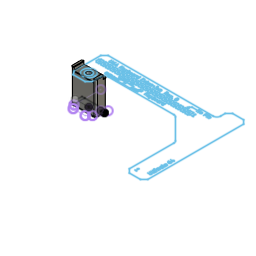
U64_KeybExt_Support v2 (Autodesk Fusion 360 design; units mm, degrees)
Autodesk Fusion 360 part; units mm, degrees
ref_plane "WorkPlane1" through (0, 0, 16) normal (0, 0, 1) x (1, 0, 0) in component "PCB"
sketch "U64_KB_Ada" plane through (0, 0, 16) normal (0, 0, 1) x (1, 0, 0) in component "PCB"
  line L0 (47.6716, 39.5) -> (12, 39.5)
  line L1 (71, 2) -> (71, 54)
  arc A0 (61, 26.1716) -> (60.4142, 27.5858) centre (59, 26.1716) ccw
  arc A1 (59, 49.5) -> (61, 51.5) centre (59, 51.5) ccw
  line L2 (71, 54) -> (69, 56)
  arc A2 (12, 39.5) -> (10, 37.5) centre (12, 37.5) ccw
  line L3 (61, 2) -> (63, 0)
  line L4 (0, 33) -> (0, 47.5)
  line L5 (61, 26.1716) -> (61, 2)
  line L6 (59, 49.5) -> (2, 49.5)
  line L7 (2, 49.5) -> (0, 47.5)
  line L8 (1.5, 31) -> (0, 33)
  line L9 (69, 0) -> (71, 2)
  line L10 (63, 0) -> (69, 0)
  line L11 (61, 54) -> (61, 51.5)
  line L12 (10, 33) -> (8, 31)
  line L13 (69, 56) -> (63, 56)
  line L14 (63, 56) -> (61, 54)
  line L15 (10, 37.5) -> (10, 33)
  line L16 (49.0858, 38.9142) -> (60.4142, 27.5858)
  arc A3 (49.0858, 38.9142) -> (47.6716, 39.5) centre (47.6716, 37.5) ccw
  line L17 (8, 31) -> (1.5, 31)
  line L18 (21.59, 45.135) -> (22.225, 45.77)
  line L19 (15.875, 43.23) -> (14.605, 43.23)
  line L20 (17.145, 45.77) -> (18.415, 45.77)
  line L21 (21.59, 45.135) -> (20.955, 45.77)
  line L22 (13.97, 45.135) -> (13.335, 45.77)
  line L23 (5.715, 43.23) -> (6.35, 43.865)
  line L24 (9.525, 43.23) -> (8.89, 43.865)
  line L25 (13.204, 40.1285) -> (13.5992, 41.215)
  line L26 (9.525, 45.77) -> (10.795, 45.77)
  line L27 (21.59, 43.865) -> (21.59, 45.135)
  line L28 (20.955, 43.23) -> (21.59, 43.865)
  line L29 (11.43, 43.865) -> (10.795, 43.23)
  line L30 (6.985, 45.77) -> (8.255, 45.77)
  line L31 (6.35, 43.865) -> (6.35, 45.135)
  line L32 (13.97, 43.865) -> (13.97, 45.135)
  line L33 (11.43, 45.135) -> (12.065, 45.77)
  line L34 (12.065, 43.23) -> (11.43, 43.865)
  circle A4 centre (5, 36) radius 3.1789
  circle A5 centre (5, 36) radius 1.7463
  line L35 (13.97, 45.135) -> (14.605, 45.77)
  line L36 (4.445, 43.23) -> (3.81, 43.865)
  line L37 (16.51, 43.865) -> (15.875, 43.23)
  line L38 (16.51, 43.865) -> (16.51, 45.135)
  line L39 (20.955, 43.23) -> (19.685, 43.23)
  line L40 (8.89, 45.135) -> (9.525, 45.77)
  line L41 (12.065, 45.77) -> (13.335, 45.77)
  line L42 (19.685, 45.77) -> (20.955, 45.77)
  line L43 (19.685, 43.23) -> (19.05, 43.865)
  line L44 (10.795, 43.23) -> (9.525, 43.23)
  line L45 (27.305, 43.23) -> (26.67, 43.865)
  line L46 (19.05, 43.865) -> (19.05, 45.135)
  line L47 (23.495, 45.77) -> (24.13, 45.135)
  line L48 (14.605, 45.77) -> (15.875, 45.77)
  line L49 (8.255, 43.23) -> (6.985, 43.23)
  line L50 (15.875, 45.77) -> (16.51, 45.135)
  line L51 (17.145, 43.23) -> (16.51, 43.865)
  line L52 (11.43, 43.865) -> (11.43, 45.135)
  line L53 (8.89, 43.865) -> (8.255, 43.23)
  line L54 (19.05, 45.135) -> (19.685, 45.77)
  line L55 (28.575, 43.23) -> (27.305, 43.23)
  line L56 (6.35, 45.135) -> (6.985, 45.77)
  line L57 (18.415, 45.77) -> (19.05, 45.135)
  line L58 (14.605, 43.23) -> (13.97, 43.865)
  line L59 (24.13, 43.865) -> (23.495, 43.23)
  line L60 (6.35, 45.135) -> (5.715, 45.77)
  line L61 (19.05, 43.865) -> (18.415, 43.23)
  line L62 (5.715, 43.23) -> (4.445, 43.23)
  line L63 (8.89, 43.865) -> (8.89, 45.135)
  line L64 (22.225, 43.23) -> (21.59, 43.865)
  line L65 (6.985, 43.23) -> (6.35, 43.865)
  line L66 (10.795, 45.77) -> (11.43, 45.135)
  line L67 (22.225, 45.77) -> (23.495, 45.77)
  line L68 (4.445, 45.77) -> (5.715, 45.77)
  line L69 (3.81, 45.135) -> (4.445, 45.77)
  line L70 (23.495, 43.23) -> (22.225, 43.23)
  arc A6 (15.2146, 40.6718) -> (15.0664, 40.82) centre (15.0664, 40.6718) ccw
  line L71 (8.255, 45.77) -> (8.89, 45.135)
  line L72 (13.335, 43.23) -> (12.065, 43.23)
  line L73 (13.335, 43.23) -> (13.97, 43.865)
  line L74 (14.8195, 40.2273) -> (14.8195, 40.8199)
  line L75 (16.51, 45.135) -> (17.145, 45.77)
  line L76 (13.96, 40.3754) -> (13.96, 40.6718)
  line L77 (12.628, 40.7211) -> (12.3317, 40.7211)
  line L78 (18.415, 43.23) -> (17.145, 43.23)
  line L79 (39.37, 45.135) -> (40.005, 45.77)
  line L80 (37.465, 43.23) -> (36.83, 43.865)
  line L81 (36.83, 45.135) -> (37.465, 45.77)
  line L82 (31.75, 43.865) -> (31.115, 43.23)
  line L83 (27.305, 45.77) -> (28.575, 45.77)
  line L84 (42.545, 43.23) -> (41.91, 43.865)
  line L85 (43.815, 43.23) -> (44.45, 43.865)
  line L86 (51.435, 43.23) -> (50.165, 43.23)
  line L87 (24.765, 43.23) -> (24.13, 43.865)
  line L88 (32.385, 45.77) -> (33.655, 45.77)
  line L89 (31.115, 43.23) -> (29.845, 43.23)
  line L90 (33.655, 43.23) -> (32.385, 43.23)
  line L91 (34.925, 45.77) -> (36.195, 45.77)
  line L92 (32.385, 43.23) -> (31.75, 43.865)
  line L93 (26.035, 45.77) -> (26.67, 45.135)
  line L94 (36.83, 43.865) -> (36.83, 45.135)
  line L95 (46.99, 43.865) -> (46.355, 43.23)
  line L96 (34.925, 43.23) -> (34.29, 43.865)
  line L97 (34.29, 43.865) -> (33.655, 43.23)
  line L98 (40.005, 43.23) -> (39.37, 43.865)
  line L99 (38.735, 45.77) -> (39.37, 45.135)
  line L100 (36.195, 43.23) -> (34.925, 43.23)
  line L101 (24.13, 45.135) -> (24.765, 45.77)
  line L102 (41.91, 45.135) -> (42.545, 45.77)
  line L103 (45.085, 43.23) -> (44.45, 43.865)
  line L104 (45.085, 45.77) -> (46.355, 45.77)
  line L105 (39.37, 43.865) -> (39.37, 45.135)
  line L106 (34.29, 43.865) -> (34.29, 45.135)
  line L107 (36.83, 45.135) -> (36.195, 45.77)
  line L108 (29.21, 45.135) -> (28.575, 45.77)
  line L109 (42.545, 45.77) -> (43.815, 45.77)
  line L110 (41.275, 43.23) -> (40.005, 43.23)
  line L111 (24.13, 43.865) -> (24.13, 45.135)
  line L112 (34.29, 45.135) -> (34.925, 45.77)
  line L113 (31.75, 45.135) -> (32.385, 45.77)
  line L114 (44.45, 43.865) -> (44.45, 45.135)
  line L115 (33.655, 45.77) -> (34.29, 45.135)
  line L116 (26.035, 43.23) -> (24.765, 43.23)
  line L117 (41.275, 45.77) -> (41.91, 45.135)
  line L118 (38.735, 43.23) -> (37.465, 43.23)
  line L119 (29.21, 43.865) -> (29.21, 45.135)
  line L120 (43.815, 43.23) -> (42.545, 43.23)
  line L121 (37.465, 45.77) -> (38.735, 45.77)
  line L122 (40.005, 45.77) -> (41.275, 45.77)
  line L123 (31.75, 43.865) -> (31.75, 45.135)
  line L124 (50.165, 43.23) -> (49.53, 43.865)
  line L125 (29.21, 45.135) -> (29.845, 45.77)
  line L126 (26.67, 43.865) -> (26.035, 43.23)
  line L127 (26.67, 43.865) -> (26.67, 45.135)
  line L128 (28.575, 43.23) -> (29.21, 43.865)
  line L129 (41.91, 43.865) -> (41.275, 43.23)
  line L130 (36.195, 43.23) -> (36.83, 43.865)
  line L131 (24.765, 45.77) -> (26.035, 45.77)
  line L132 (29.845, 45.77) -> (31.115, 45.77)
  line L133 (46.355, 43.23) -> (45.085, 43.23)
  line L134 (44.45, 45.135) -> (43.815, 45.77)
  line L135 (3.81, 43.865) -> (3.81, 45.135)
  line L136 (46.355, 45.77) -> (46.99, 45.135)
  line L137 (44.45, 45.135) -> (45.085, 45.77)
  line L138 (49.53, 43.865) -> (49.53, 45.135)
  line L139 (31.115, 45.77) -> (31.75, 45.135)
  line L140 (26.67, 45.135) -> (27.305, 45.77)
  line L141 (41.91, 43.865) -> (41.91, 45.135)
  line L142 (29.845, 43.23) -> (29.21, 43.865)
  line L143 (16.0338, 40.0685) -> (16.4148, 40.0685)
  line L144 (15.5258, 40.0304) -> (15.5258, 41.8846)
  line L145 (46.99, 43.865) -> (46.99, 45.135)
  line L146 (3.81, 45.135) -> (3.175, 45.77)
  line L147 (3.175, 43.23) -> (3.81, 43.865)
  line L148 (47.625, 43.23) -> (46.99, 43.865)
  line L149 (19.812, 41.8846) -> (19.812, 40.0304)
  line L150 (16.4148, 40.0685) -> (16.4148, 40.1955)
  line L151 (51.435, 43.23) -> (52.07, 43.865)
  line L152 (39.37, 43.865) -> (38.735, 43.23)
  line L153 (48.895, 45.77) -> (49.53, 45.135)
  line L154 (16.4148, 41.8465) -> (16.0338, 41.8465)
  line L155 (23.368, 41.8846) -> (23.368, 40.0304)
  line L156 (19.812, 41.8846) -> (23.368, 41.8846)
  line L157 (16.1608, 40.0304) -> (15.5258, 40.0304)
  line L158 (16.0338, 41.7195) -> (16.4148, 41.7195)
  line L159 (46.99, 45.135) -> (47.625, 45.77)
  line L160 (49.53, 43.865) -> (48.895, 43.23)
  line L161 (49.53, 45.135) -> (50.165, 45.77)
  line L162 (19.0817, 40.0304) -> (19.0817, 41.8846)
  line L163 (47.625, 45.77) -> (48.895, 45.77)
  line L164 (16.0338, 41.8465) -> (16.0338, 41.7195)
  line L165 (15.5258, 41.8846) -> (19.0817, 41.8846)
  line L166 (52.07, 45.135) -> (52.07, 45.77)
  line L167 (48.895, 43.23) -> (47.625, 43.23)
  line L168 (1.27, 43.865) -> (1.27, 45.135)
  line L169 (19.0817, 40.0304) -> (16.1608, 40.0304)
  line L170 (16.4148, 41.7195) -> (16.4148, 41.8465)
  line L171 (23.368, 40.0304) -> (19.812, 40.0304)
  line L172 (1.905, 45.77) -> (3.175, 45.77)
  line L173 (1.27, 45.135) -> (1.905, 45.77)
  line L174 (52.07, 43.865) -> (52.07, 45.135)
  line L175 (16.4148, 40.1955) -> (16.0338, 40.1955)
  line L176 (50.165, 45.77) -> (52.07, 45.77)
  line L177 (1.905, 43.23) -> (1.27, 43.865)
  line L178 (3.175, 43.23) -> (1.905, 43.23)
  line L179 (16.0338, 40.1955) -> (16.0338, 40.0685)
  line L180 (36.7207, 46.8778) -> (36.7207, 47.3153)
  line L181 (32.2069, 46.6153) -> (32.2069, 47.6652)
  arc A7 (30.8, 46.9653) -> (31.5, 46.9653) centre (31.15, 46.9653) ccw
  line L182 (32.2069, 47.6652) -> (32.6443, 47.6652)
  line L183 (32.9068, 47.4028) -> (32.9068, 46.6153)
  line L184 (37.4206, 46.6153) -> (36.9832, 46.6153)
  arc A8 (32.9068, 47.4028) -> (32.6443, 47.6653) centre (32.6443, 47.4028) ccw
  line L185 (35.1853, 46.6153) -> (35.1853, 48.1902)
  arc A9 (31.5, 47.3153) -> (30.8, 47.3153) centre (31.15, 47.3153) ccw
  line L186 (31.5, 47.3153) -> (31.5, 46.9653)
  line L187 (36.0602, 46.6153) -> (35.7103, 47.3153)
  arc A10 (36.7207, 46.8778) -> (36.9832, 46.6153) centre (36.9832, 46.8778) ccw
  line L188 (68.0149, 5.0229) -> (69.1522, 5.0229)
  line L189 (68.0149, 7.4951) -> (69.3272, 7.4951)
  line L190 (48.26, 47.1487) -> (49.0538, 47.9425)
  arc A11 (68.9772, 11.2434) -> (69.5896, 11.2434) centre (69.2834, 11.2434) ccw
  line L191 (32.8769, 40.5342) -> (33.0518, 40.5342)
  arc A12 (68.8022, 10.2057) -> (68.5397, 9.9432) centre (68.8022, 9.9432) ccw
  line L192 (32.2742, 41.584) -> (31.5743, 41.584)
  line L193 (68.9772, 11.6371) -> (68.9772, 11.2434)
  line L194 (30.9802, 42.6339) -> (30.1054, 41.6715)
  arc A13 (37.6321, 41.8465) -> (37.3696, 42.109) centre (37.3696, 41.8465) ccw
  line L195 (49.0538, 47.9425) -> (51.5938, 47.9425)
  arc A14 (68.8897, 14.0427) -> (68.8897, 13.3427) centre (68.8897, 13.6927) ccw
  arc A15 (37.2384, 41.6715) -> (37.2384, 41.0591) centre (37.2384, 41.3653) ccw
  line L196 (68.0149, 8.474) -> (68.1023, 8.474)
  line L197 (39.4332, 41.3216) -> (39.4332, 41.8465)
  line L198 (68.5398, 12.2179) -> (68.5398, 12.7428)
  arc A16 (34.6778, 41.0591) -> (34.9403, 41.3216) centre (34.6778, 41.3216) ccw
  line L199 (37.6321, 41.6715) -> (37.2384, 41.6715)
  line L200 (30.9802, 41.0591) -> (30.4553, 42.0215)
  line L201 (40.1331, 41.0591) -> (39.6956, 41.0591)
  line L202 (35.1853, 48.1902) -> (35.6228, 48.1902)
  line L203 (37.6321, 41.0591) -> (37.6321, 41.8465)
  line L204 (69.5897, 11.2434) -> (69.5897, 11.6371)
  line L205 (34.2404, 42.6339) -> (34.2404, 41.0591)
  line L206 (69.0647, 14.0427) -> (69.0647, 13.3428)
  line L207 (38.4101, 42.109) -> (38.935, 42.109)
  line L208 (31.5743, 41.3216) -> (31.5743, 41.759)
  arc A17 (32.2742, 41.759) -> (31.5742, 41.759) centre (31.9242, 41.759) ccw
  arc A18 (35.6228, 47.3153) -> (35.6228, 48.1901) centre (35.6228, 47.7527) ccw
  arc A19 (31.5742, 41.3216) -> (31.8367, 41.0591) centre (31.8367, 41.3216) ccw
  line L209 (32.8769, 42.109) -> (33.2268, 41.0591)
  line L210 (68.8897, 14.0427) -> (69.0647, 14.0427)
  line L211 (39.6956, 42.109) -> (40.1331, 42.109)
  arc A20 (69.3272, 13.3427) -> (69.5897, 13.6052) centre (69.3272, 13.6052) ccw
  line L212 (32.2742, 41.759) -> (32.2742, 41.584)
  arc A21 (39.4331, 41.3216) -> (39.6956, 41.0591) centre (39.6956, 41.3216) ccw
  line L213 (68.7148, 15.5479) -> (68.7148, 16.0728)
  arc A22 (69.0647, 16.4228) -> (68.7147, 16.0728) centre (69.0647, 16.0728) ccw
  line L214 (30.1054, 41.0591) -> (30.1054, 42.6339)
  line L215 (35.5863, 41.4091) -> (35.5863, 41.759)
  line L216 (48.26, 46.1962) -> (47.7838, 46.6725)
  line L217 (69.5897, 14.0427) -> (69.5897, 13.6052)
  line L218 (35.6228, 47.3153) -> (35.1853, 47.3153)
  line L219 (69.5897, 12.6553) -> (69.5897, 12.7428)
  line L220 (68.5398, 9.1558) -> (68.5398, 9.9432)
  line L221 (32.2742, 41.0591) -> (31.8367, 41.0591)
  arc A23 (68.8023, 11.6371) -> (68.5398, 11.3746) centre (68.8023, 11.3746) ccw
  line L222 (69.5897, 11.6371) -> (68.8023, 11.6371)
  line L223 (68.8023, 10.2057) -> (69.5897, 10.2057)
  line L224 (48.26, 46.1962) -> (48.26, 47.1487)
  line L225 (69.5897, 9.6807) -> (68.5398, 9.6807)
  line L226 (69.5897, 8.4302) -> (68.5398, 8.4302)
  line L227 (68.1023, 8.3865) -> (68.0149, 8.3865)
  line L228 (48.26, 46.1962) -> (48.7363, 46.6725)
  line L229 (11.7091, 46.6153) -> (11.1842, 47.5777)
  line L230 (68.0149, 12.3929) -> (69.3272, 12.3929)
  arc A24 (69.3272, 7.4951) -> (69.5897, 7.7576) centre (69.3272, 7.7576) ccw
  line L231 (36.2862, 41.759) -> (36.2862, 41.4091)
  line L232 (33.0518, 40.5342) -> (33.5768, 42.109)
  arc A25 (36.2862, 41.759) -> (35.5862, 41.759) centre (35.9362, 41.759) ccw
  line L233 (57.4631, 48.7377) -> (57.4631, 48.8252)
  line L234 (69.1522, 5.8977) -> (68.0149, 5.8977)
  arc A26 (56.4901, 47.9503) -> (56.4901, 48.8251) centre (56.4901, 48.3877) ccw
  arc A27 (58.8989, 48.0378) -> (58.6364, 48.3003) centre (58.6364, 48.0378) ccw
  line L235 (6.7968, 47.0528) -> (6.7968, 47.4902)
  line L236 (8.9724, 47.3153) -> (8.9724, 46.6153)
  arc A28 (12.3031, 46.8778) -> (12.5656, 46.6153) centre (12.5656, 46.8778) ccw
  line L237 (6.7968, 47.4902) -> (7.3218, 47.4902)
  line L238 (69.5897, 7.7576) -> (69.5897, 7.845)
  line L239 (68.0149, 8.3865) -> (68.0149, 8.474)
  line L240 (40.1331, 42.6339) -> (40.1331, 41.0591)
  line L241 (38.4101, 41.0591) -> (38.4101, 42.109)
  line L242 (68.0149, 6.6393) -> (69.3272, 6.6393)
  line L243 (8.36, 46.9653) -> (9.2348, 46.9653)
  line L244 (54.47, 47.9503) -> (54.47, 47.6003)
  arc A29 (34.9403, 41.8465) -> (34.6778, 42.109) centre (34.6778, 41.8465) ccw
  line L245 (56.4901, 47.9503) -> (56.0527, 47.9503)
  line L246 (13.0031, 46.6153) -> (12.5656, 46.6153)
  line L247 (53.0465, 47.2504) -> (53.0465, 48.8252)
  line L248 (12.3031, 46.8778) -> (12.3031, 47.3153)
  line L249 (34.9403, 41.3216) -> (34.9403, 41.8465)
  line L250 (69.1522, 15.5479) -> (68.7148, 15.5479)
  arc A30 (35.5862, 41.4091) -> (36.2862, 41.4091) centre (35.9362, 41.4091) ccw
  line L251 (56.0527, 48.8252) -> (56.4901, 48.8252)
  line L252 (68.1023, 8.474) -> (68.1023, 8.3865)
  arc A31 (69.1522, 5.0229) -> (69.1522, 5.8977) centre (69.1522, 5.4603) ccw
  arc A32 (13.0031, 47.3153) -> (12.3031, 47.3153) centre (12.6531, 47.3153) ccw
  arc A33 (69.3272, 6.6392) -> (69.5897, 6.9017) centre (69.3272, 6.9017) ccw
  line L253 (38.935, 42.109) -> (38.935, 41.934)
  arc A34 (39.6956, 42.109) -> (39.4331, 41.8465) centre (39.6956, 41.8465) ccw
  line L254 (69.5897, 9.1558) -> (68.5398, 9.1558)
  line L255 (11.7091, 48.1902) -> (10.8342, 47.2278)
  line L256 (63.1254, 4.1839) -> (63.5628, 4.5339)
  line L257 (68.5398, 11.3746) -> (68.5398, 11.0247)
  arc A35 (69.3272, 12.3928) -> (69.5897, 12.6553) centre (69.3272, 12.6553) ccw
  line L258 (37.2384, 41.0591) -> (37.6321, 41.0591)
  line L259 (34.2404, 41.0591) -> (34.6778, 41.0591)
  line L260 (69.3272, 13.3428) -> (68.8897, 13.3428)
  line L261 (6.0565, 47.0528) -> (6.0565, 48.1902)
  line L262 (7.6717, 47.1403) -> (7.6717, 47.0528)
  line L263 (52.1716, 47.2504) -> (52.1716, 48.8252)
  arc A36 (5.1816, 47.0528) -> (6.0564, 47.0528) centre (5.619, 47.0528) ccw
  line L264 (68.5398, 7.3201) -> (68.5398, 7.845)
  line L265 (15.4067, 47.6652) -> (14.9693, 47.6652)
  line L266 (13.0031, 47.1403) -> (12.3031, 47.1403)
  line L267 (37.3696, 42.109) -> (37.0197, 42.109)
  arc A37 (54.4701, 47.9503) -> (53.7701, 47.9503) centre (54.1201, 47.9503) ccw
  line L268 (58.199, 48.3002) -> (58.6364, 48.3002)
  line L269 (34.6778, 42.109) -> (34.2404, 42.109)
  line L270 (57.5068, 47.2504) -> (57.5068, 48.3002)
  line L271 (52.9654, 43.9166) -> (53.8402, 43.9166)
  line L272 (27.4133, 47.6652) -> (27.8508, 47.6652)
  line L273 (8.7099, 48.1902) -> (8.36, 46.9653)
  line L274 (13.6057, 46.0904) -> (13.7807, 46.0904)
  arc A38 (7.4967, 48.1901) -> (6.7968, 47.4902) centre (7.4967, 47.4902) ccw
  line L275 (15.6692, 46.8778) -> (15.6692, 47.4028)
  line L276 (5.1816, 48.1902) -> (5.1816, 47.0528)
  arc A39 (17.0151, 47.3153) -> (16.3151, 47.3153) centre (16.6651, 47.3153) ccw
  arc A40 (53.7701, 47.6003) -> (54.4701, 47.6003) centre (54.1201, 47.6003) ccw
  line L277 (20.862, 46.6153) -> (20.4245, 46.6153)
  arc A41 (69.1522, 15.5479) -> (69.1522, 16.4227) centre (69.1522, 15.9853) ccw
  line L278 (30.1163, 48.1027) -> (30.1163, 48.1902)
  line L279 (13.0031, 47.3153) -> (13.0031, 47.1403)
  line L280 (26.0065, 46.8778) -> (26.0065, 47.3153)
  line L281 (30.1163, 48.1902) -> (30.2038, 48.1902)
  line L282 (19.139, 47.6652) -> (19.6639, 47.6652)
  line L283 (52.1716, 48.8252) -> (53.0465, 47.2504)
  arc A42 (68.0149, 16.2478) -> (68.7148, 15.5479) centre (68.7148, 16.2478) ccw
  arc A43 (15.6692, 47.4028) -> (15.4067, 47.6653) centre (15.4067, 47.4028) ccw
  arc A44 (17.9673, 47.2278) -> (17.9673, 46.6154) centre (17.9673, 46.9216) ccw
  line L284 (22.4837, 47.4902) -> (23.0087, 47.4902)
  line L285 (53.4028, 45.4914) -> (53.4028, 43.9166)
  arc A45 (29.4325, 47.5777) -> (29.0388, 47.6652) centre (29.0246, 46.6717) ccw
  line L286 (52.9654, 45.1414) -> (53.4028, 45.4914)
  line L287 (26.7064, 47.1403) -> (26.0065, 47.1403)
  arc A46 (28.1133, 47.4028) -> (27.8508, 47.6653) centre (27.8508, 47.4028) ccw
  arc A47 (7.6718, 47.1403) -> (7.3218, 47.4903) centre (7.3218, 47.1403) ccw
  arc A48 (15.4067, 46.6153) -> (15.6692, 46.8778) centre (15.4067, 46.8778) ccw
  arc A49 (28.8201, 46.7028) -> (29.3013, 46.6154) centre (29.3225, 48.0991) ccw
  arc A50 (18.361, 47.4028) -> (18.0985, 47.6653) centre (18.0985, 47.4028) ccw
  line L288 (57.5506, 48.8252) -> (57.5506, 48.7377)
  arc A51 (25.0566, 46.8778) -> (25.3191, 46.6153) centre (25.3191, 46.8778) ccw
  line L289 (18.361, 47.2278) -> (17.9673, 47.2278)
  line L290 (25.3191, 46.6153) -> (25.4066, 46.6153)
  line L291 (10.8342, 46.6153) -> (10.8342, 48.1902)
  line L292 (30.2038, 48.1902) -> (30.2038, 48.1027)
  line L293 (16.3152, 46.9653) -> (16.3152, 47.3153)
  line L294 (30.2038, 48.1027) -> (30.1163, 48.1027)
  line L295 (30.8001, 46.9653) -> (30.8001, 47.3153)
  line L296 (22.4837, 48.1902) -> (23.1837, 48.1902)
  line L297 (58.8989, 48.0378) -> (58.8989, 47.2504)
  line L298 (13.6057, 47.6652) -> (13.9557, 46.6153)
  line L299 (63.5628, 4.5339) -> (63.5628, 2.9591)
  line L300 (18.361, 46.6153) -> (18.361, 47.4028)
  line L301 (57.4631, 48.8252) -> (57.5506, 48.8252)
  line L302 (68.0149, 17.4609) -> (69.2397, 17.111)
  line L303 (56.0527, 47.2504) -> (56.0527, 48.8252)
  line L304 (69.0647, 16.4228) -> (69.1522, 16.4228)
  line L305 (14.9693, 46.6153) -> (15.4067, 46.6153)
  line L306 (53.7701, 47.6003) -> (53.7701, 47.9503)
  line L307 (13.7807, 46.0904) -> (14.3057, 47.6652)
  arc A52 (26.7065, 47.3153) -> (26.0065, 47.3153) centre (26.3565, 47.3153) ccw
  line L308 (30.1601, 46.6153) -> (30.1601, 47.6652)
  line L309 (23.1837, 46.6153) -> (22.4837, 46.6153)
  arc A53 (20.162, 46.8778) -> (20.4245, 46.6153) centre (20.4245, 46.8778) ccw
  line L310 (14.9693, 48.1902) -> (14.9693, 46.6153)
  line L311 (63.1254, 2.9591) -> (64.0002, 2.9591)
  line L312 (69.2397, 17.111) -> (69.2397, 17.9859)
  line L313 (20.162, 46.8778) -> (20.162, 47.4028)
  arc A54 (6.7969, 47.0528) -> (7.6717, 47.0528) centre (7.2343, 47.0528) ccw
  line L314 (58.199, 47.2504) -> (58.199, 48.3002)
  line L315 (68.8897, 17.7234) -> (69.5897, 17.7234)
  line L316 (17.0151, 47.3153) -> (17.0151, 46.9653)
  line L317 (57.5506, 48.7377) -> (57.4631, 48.7377)
  arc A55 (11.4914, 40.3507) -> (11.6642, 40.2273) centre (11.6642, 40.41) ccw
  arc A56 (11.837, 40.9927) -> (11.6642, 41.1162) centre (11.6642, 40.9335) ccw
  line L318 (40.8891, 46.9653) -> (41.589, 47.8402)
  arc A57 (10.5522, 40.9187) -> (10.9474, 40.9187) centre (10.7498, 40.9187) ccw
  line L319 (29.3888, 47.0528) -> (28.9514, 47.2278)
  line L320 (22.4837, 46.6153) -> (22.4837, 48.1902)
  arc A58 (25.9658, 40.9927) -> (25.793, 41.1162) centre (25.793, 40.9335) ccw
  line L321 (26.7064, 46.6153) -> (26.269, 46.6153)
  line L322 (39.3549, 46.7028) -> (39.3549, 46.6153)
  arc A59 (9.6626, 40.9928) -> (9.5885, 40.6718) centre (10.3211, 40.6718) ccw
  arc A60 (40.8015, 47.4028) -> (40.9327, 46.8341) centre (42.0993, 47.4028) ccw
  arc A61 (23.9642, 40.2273) -> (23.9642, 40.7211) centre (23.9642, 40.4742) ccw
  line L323 (39.2674, 46.6153) -> (39.2674, 46.7028)
  line L324 (26.4985, 40.2273) -> (26.4985, 41.1163)
  arc A62 (10.9967, 40.4742) -> (10.5029, 40.4742) centre (10.7498, 40.4742) ccw
  line L325 (25.0566, 48.1902) -> (25.0566, 46.8778)
  line L326 (23.7139, 47.6652) -> (24.4138, 46.6153)
  arc A63 (16.3151, 46.9653) -> (17.0151, 46.9653) centre (16.6651, 46.9653) ccw
  line L327 (38.3733, 46.6153) -> (38.7232, 47.6652)
  line L328 (24.8816, 47.6652) -> (25.4066, 47.6652)
  line L329 (26.7454, 40.6224) -> (26.4985, 40.6224)
  line L330 (20.4245, 47.6652) -> (20.862, 47.6652)
  arc A64 (9.8354, 41.1162) -> (9.6626, 40.9928) centre (9.8354, 40.9335) ccw
  line L331 (19.139, 46.6153) -> (19.139, 47.6652)
  arc A65 (29.3014, 46.6154) -> (29.3888, 47.0528) centre (29.3046, 46.8422) ccw
  arc A66 (26.0065, 46.8778) -> (26.269, 46.6153) centre (26.269, 46.8778) ccw
  line L332 (26.7064, 47.3153) -> (26.7064, 47.1403)
  arc A67 (25.793, 41.1162) -> (25.6202, 40.9928) centre (25.793, 40.9335) ccw
  arc A68 (41.239, 46.6154) -> (41.5452, 46.8341) centre (41.239, 46.9391) ccw
  arc A69 (10.0082, 40.9927) -> (9.8354, 41.1162) centre (9.8354, 40.9335) ccw
  arc A70 (24.928, 40.7211) -> (24.928, 41.1163) centre (24.928, 40.9187) ccw
  arc A71 (24.8786, 40.2273) -> (24.8786, 40.7211) centre (24.8786, 40.4742) ccw
  line L333 (26.4985, 41.1163) -> (26.7454, 41.1163)
  line L334 (9.6379, 40.4248) -> (10.033, 40.9187)
  line L335 (26.9924, 40.2273) -> (26.7948, 40.6224)
  arc A72 (9.6626, 40.3507) -> (9.8354, 40.2273) centre (9.8354, 40.41) ccw
  line L336 (20.862, 48.1902) -> (20.862, 46.6153)
  line L337 (18.0985, 47.6652) -> (17.7485, 47.6652)
  arc A73 (29.0388, 47.6652) -> (28.9514, 47.2278) centre (29.0356, 47.4384) ccw
  line L338 (24.928, 40.7211) -> (24.7304, 40.7211)
  arc A74 (11.9112, 40.6718) -> (11.8371, 40.9928) centre (11.1786, 40.6718) ccw
  line L339 (23.7172, 40.2273) -> (23.9642, 40.2273)
  line L340 (37.4206, 47.1403) -> (36.7207, 47.1403)
  line L341 (27.4133, 46.6153) -> (27.4133, 47.6652)
  line L342 (39.3549, 46.6153) -> (39.2674, 46.6153)
  line L343 (17.9673, 46.6153) -> (18.361, 46.6153)
  line L344 (28.1132, 47.4028) -> (28.1132, 46.6153)
  arc A75 (24.0136, 40.7211) -> (24.0136, 41.1163) centre (24.0136, 40.9187) ccw
  arc A76 (41.5452, 47.9714) -> (41.239, 48.1901) centre (41.239, 47.8664) ccw
  arc A77 (20.4245, 47.6653) -> (20.162, 47.4028) centre (20.4245, 47.4028) ccw
  line L345 (24.6317, 40.2273) -> (24.8786, 40.2273)
  line L346 (23.7172, 41.1163) -> (24.0136, 41.1163)
  arc A78 (11.4914, 40.9928) -> (11.4173, 40.6718) centre (12.1499, 40.6718) ccw
  arc A79 (25.5461, 40.6718) -> (25.6202, 40.3508) centre (26.2787, 40.6718) ccw
  arc A80 (10.5029, 40.4742) -> (10.9967, 40.4742) centre (10.7498, 40.4742) ccw
  arc A81 (11.6642, 41.1162) -> (11.4914, 40.9928) centre (11.6642, 40.9335) ccw
  line L347 (24.0136, 40.7211) -> (23.816, 40.7211)
  arc A82 (11.8371, 40.3508) -> (11.9112, 40.6718) centre (11.1786, 40.6718) ccw
  arc A83 (25.6202, 40.3507) -> (25.793, 40.2273) centre (25.793, 40.41) ccw
  arc A84 (25.9658, 40.3508) -> (26.0399, 40.6718) centre (25.3073, 40.6718) ccw
  line L348 (23.7139, 46.6153) -> (24.4138, 47.6652)
  arc A85 (11.4173, 40.6718) -> (11.4914, 40.3508) centre (12.1499, 40.6718) ccw
  line L349 (19.6639, 47.6652) -> (19.6639, 47.4902)
  arc A86 (25.793, 40.2273) -> (25.9658, 40.3507) centre (25.793, 40.41) ccw
  arc A87 (12.628, 40.2272) -> (12.8256, 40.4248) centre (12.628, 40.4248) ccw
  line L350 (12.3317, 40.7211) -> (12.3317, 41.1163)
  line L351 (14.8273, 42.6367) -> (15.4199, 42.6367)
  arc A88 (13.96, 40.3754) -> (14.1082, 40.2272) centre (14.1082, 40.3754) ccw
  line L352 (19.4098, 42.3404) -> (19.4098, 42.9331)
  arc A89 (9.5885, 40.6718) -> (9.6626, 40.3508) centre (10.3211, 40.6718) ccw
  line L353 (19.1135, 42.6367) -> (19.7062, 42.6367)
  line L354 (14.3551, 40.8199) -> (14.3551, 40.0791)
  line L355 (14.207, 39.9309) -> (14.0094, 39.9309)
  line L356 (39.2674, 46.7028) -> (39.3549, 46.7028)
  line L357 (25.5954, 40.4248) -> (25.9906, 40.9187)
  arc A90 (26.7454, 40.6224) -> (26.7454, 41.1162) centre (26.7454, 40.8693) ccw
  line L358 (38.0233, 47.6652) -> (38.3733, 46.6153)
  arc A91 (41.239, 48.1901) -> (40.9328, 47.9714) centre (41.239, 47.8664) ccw
  arc A92 (41.6764, 47.4028) -> (41.5452, 47.9715) centre (40.3787, 47.4028) ccw
  arc A93 (9.8354, 40.2273) -> (10.0082, 40.3507) centre (9.8354, 40.41) ccw
  line L359 (11.4667, 40.4248) -> (11.8618, 40.9187)
  line L360 (12.8256, 40.4248) -> (12.8256, 40.5236)
  arc A94 (41.5453, 46.8341) -> (41.6765, 47.4028) centre (40.3787, 47.4028) ccw
  arc A95 (11.6642, 40.2273) -> (11.837, 40.3507) centre (11.6642, 40.41) ccw
  line L361 (37.4206, 47.3153) -> (37.4206, 47.1403)
  arc A96 (14.1082, 40.82) -> (13.96, 40.6718) centre (14.1082, 40.6718) ccw
  arc A97 (14.2069, 39.9309) -> (14.3551, 40.0791) centre (14.2069, 40.0791) ccw
  line L362 (15.2146, 40.6718) -> (15.2146, 40.2273)
  line L363 (14.1082, 40.8199) -> (14.3551, 40.8199)
  arc A98 (40.9328, 46.8341) -> (41.239, 46.6154) centre (41.239, 46.9391) ccw
  line L364 (12.3317, 40.2273) -> (12.628, 40.2273)
  arc A99 (37.4207, 47.3153) -> (36.7207, 47.3153) centre (37.0707, 47.3153) ccw
  arc A100 (12.8256, 40.5236) -> (12.628, 40.7212) centre (12.628, 40.5236) ccw
  arc A101 (10.0083, 40.3508) -> (10.0824, 40.6718) centre (9.3498, 40.6718) ccw
  arc A102 (40.9327, 47.9715) -> (40.8015, 47.4028) centre (42.0993, 47.4028) ccw
  line L365 (12.3317, 41.1163) -> (12.8256, 41.1163)
  line L366 (24.6317, 41.1163) -> (24.928, 41.1163)
  arc A103 (26.04, 40.6718) -> (25.9659, 40.9928) centre (25.3074, 40.6718) ccw
  arc A104 (10.0824, 40.6718) -> (10.0083, 40.9928) centre (9.3498, 40.6718) ccw
  arc A105 (25.6202, 40.9928) -> (25.5461, 40.6718) centre (26.2787, 40.6718) ccw
  arc A106 (10.9474, 40.9187) -> (10.5522, 40.9187) centre (10.7498, 40.9187) ccw
  line L367 (14.3551, 40.2273) -> (14.1082, 40.2273)
  line L368 (14.8195, 40.8199) -> (15.0664, 40.8199)
  line L369 (38.354, 44.754) -> (37.846, 44.754)
  line L370 (12.446, 44.246) -> (12.954, 44.246)
  line L371 (5.334, 44.754) -> (4.826, 44.754)
  line L372 (9.906, 44.246) -> (10.414, 44.246)
  line L373 (9.906, 44.754) -> (9.906, 44.246)
  line L374 (4.826, 44.246) -> (5.334, 44.246)
  line L375 (15.494, 44.754) -> (14.986, 44.754)
  line L376 (7.366, 44.754) -> (7.366, 44.246)
  line L377 (7.874, 44.754) -> (7.366, 44.754)
  line L378 (22.606, 44.754) -> (22.606, 44.246)
  line L379 (7.874, 44.246) -> (7.874, 44.754)
  line L380 (12.954, 44.754) -> (12.446, 44.754)
  line L381 (17.526, 44.754) -> (17.526, 44.246)
  line L382 (17.526, 44.246) -> (18.034, 44.246)
  line L383 (12.954, 44.246) -> (12.954, 44.754)
  line L384 (23.114, 44.246) -> (23.114, 44.754)
  line L385 (7.366, 44.246) -> (7.874, 44.246)
  line L386 (15.494, 44.246) -> (15.494, 44.754)
  line L387 (20.574, 44.246) -> (20.574, 44.754)
  line L388 (5.334, 44.246) -> (5.334, 44.754)
  line L389 (18.034, 44.754) -> (17.526, 44.754)
  line L390 (25.146, 44.754) -> (25.146, 44.246)
  line L391 (25.146, 44.246) -> (25.654, 44.246)
  line L392 (22.606, 44.246) -> (23.114, 44.246)
  line L393 (20.574, 44.754) -> (20.066, 44.754)
  line L394 (14.986, 44.246) -> (15.494, 44.246)
  line L395 (25.654, 44.246) -> (25.654, 44.754)
  line L396 (4.826, 44.754) -> (4.826, 44.246)
  line L397 (20.066, 44.246) -> (20.574, 44.246)
  line L398 (10.414, 44.246) -> (10.414, 44.754)
  line L399 (14.986, 44.754) -> (14.986, 44.246)
  line L400 (25.654, 44.754) -> (25.146, 44.754)
  line L401 (12.446, 44.754) -> (12.446, 44.246)
  line L402 (10.414, 44.754) -> (9.906, 44.754)
  line L403 (20.066, 44.754) -> (20.066, 44.246)
  line L404 (18.034, 44.246) -> (18.034, 44.754)
  line L405 (23.114, 44.754) -> (22.606, 44.754)
  line L406 (2.794, 44.754) -> (2.286, 44.754)
  line L407 (2.286, 44.246) -> (2.794, 44.246)
  line L408 (33.274, 44.246) -> (33.274, 44.754)
  line L409 (28.194, 44.754) -> (27.686, 44.754)
  line L410 (43.434, 44.246) -> (43.434, 44.754)
  line L411 (45.466, 44.754) -> (45.466, 44.246)
  line L412 (45.974, 44.754) -> (45.466, 44.754)
  line L413 (38.354, 44.246) -> (38.354, 44.754)
  line L414 (2.794, 44.246) -> (2.794, 44.754)
  line L415 (48.514, 44.754) -> (48.006, 44.754)
  line L416 (48.006, 44.246) -> (48.514, 44.246)
  line L417 (28.194, 44.246) -> (28.194, 44.754)
  line L418 (35.814, 44.754) -> (35.306, 44.754)
  line L419 (43.434, 44.754) -> (42.926, 44.754)
  line L420 (27.686, 44.754) -> (27.686, 44.246)
  line L421 (33.274, 44.754) -> (32.766, 44.754)
  line L422 (40.894, 44.246) -> (40.894, 44.754)
  line L423 (37.846, 44.754) -> (37.846, 44.246)
  line L424 (27.686, 44.246) -> (28.194, 44.246)
  line L425 (42.926, 44.246) -> (43.434, 44.246)
  line L426 (50.546, 44.246) -> (51.054, 44.246)
  line L427 (40.386, 44.246) -> (40.894, 44.246)
  line L428 (2.286, 44.754) -> (2.286, 44.246)
  line L429 (30.734, 44.754) -> (30.226, 44.754)
  line L430 (32.766, 44.246) -> (33.274, 44.246)
  line L431 (37.846, 44.246) -> (38.354, 44.246)
  line L432 (35.814, 44.246) -> (35.814, 44.754)
  line L433 (50.546, 44.754) -> (50.546, 44.246)
  line L434 (45.974, 44.246) -> (45.974, 44.754)
  line L435 (51.054, 44.246) -> (51.054, 44.754)
  line L436 (48.006, 44.754) -> (48.006, 44.246)
  line L437 (30.734, 44.246) -> (30.734, 44.754)
  line L438 (30.226, 44.754) -> (30.226, 44.246)
  line L439 (32.766, 44.754) -> (32.766, 44.246)
  line L440 (40.894, 44.754) -> (40.386, 44.754)
  line L441 (42.926, 44.754) -> (42.926, 44.246)
  line L442 (35.306, 44.754) -> (35.306, 44.246)
  line L443 (51.054, 44.754) -> (50.546, 44.754)
  line L444 (16.4148, 41.7195) -> (16.0338, 41.7195)
  line L445 (45.466, 44.246) -> (45.974, 44.246)
  line L446 (48.514, 44.246) -> (48.514, 44.754)
  line L447 (16.0338, 40.1955) -> (16.4148, 40.1955)
  line L448 (16.4148, 40.1955) -> (16.4148, 41.7195)
  line L449 (35.306, 44.246) -> (35.814, 44.246)
  line L450 (40.386, 44.754) -> (40.386, 44.246)
  line L451 (30.226, 44.246) -> (30.734, 44.246)
  line L452 (16.0338, 41.7195) -> (16.0338, 40.1955)
  line L453 (26.7889, 42.6204) -> (26.7889, 41.7116)
  line L454 (17.129, 42.0243) -> (17.129, 42.9387)
  arc A107 (27.6733, 42.6204) -> (27.3163, 42.3607) centre (27.6733, 42.2451) ccw
  arc A108 (27.8681, 42.1011) -> (27.9655, 42.3283) centre (27.6517, 42.3283) ccw
  arc A109 (26.5293, 41.452) -> (26.7889, 41.7116) centre (26.5293, 41.7116) ccw
  line L455 (26.5293, 41.452) -> (26.3995, 41.452)
  line L456 (27.868, 42.1011) -> (27.3163, 41.452)
  line L457 (27.3163, 41.452) -> (27.9654, 41.452)
  arc A110 (27.9654, 42.3283) -> (27.6733, 42.6204) centre (27.6733, 42.3283) ccw
  line L458 (17.637, 42.6847) -> (17.637, 42.2783)
  arc A111 (17.383, 42.0243) -> (17.637, 42.2783) centre (17.383, 42.2783) ccw
  line L459 (22.0088, 42.0243) -> (22.5168, 42.0243)
  line L460 (22.0088, 42.7355) -> (22.2628, 42.9387)
  line L461 (18.0739, 42.7355) -> (18.3279, 42.9387)
  line L462 (17.129, 42.9387) -> (17.383, 42.9387)
  line L463 (21.609, 42.0243) -> (21.4059, 42.4307)
  line L464 (22.2628, 42.9387) -> (22.2628, 42.0243)
  line L465 (21.3551, 42.4307) -> (21.1011, 42.4307)
  line L466 (18.3279, 42.9387) -> (18.3279, 42.0243)
  arc A112 (17.637, 42.6847) -> (17.383, 42.9387) centre (17.383, 42.6847) ccw
  line L467 (18.0739, 42.0243) -> (18.5819, 42.0243)
  line L468 (21.1011, 42.9387) -> (21.3551, 42.9387)
  line L469 (21.1011, 42.0243) -> (21.1011, 42.9387)
  line L470 (16.3386, 42.9387) -> (16.3386, 42.0243)
  arc A113 (21.3551, 42.4307) -> (21.3551, 42.9387) centre (21.3551, 42.6847) ccw
  line L471 (16.3386, 42.0243) -> (16.7449, 42.0243)
  line L472 (17.383, 42.0243) -> (17.129, 42.0243)
sketch "base" plane through (0, 0, 0) normal (0, 0, 1) x (1, 0, 0) in component "U64_KeybExt_StandOff"
  circle A0 centre (5, 36) radius 1.7463 construction
  line L0 (0, 33) -> (0, 47.5) construction
  line L1 (1.5, 31) -> (0, 33) construction
  line L2 (8, 31) -> (1.5, 31) construction
  line L3 (10, 33) -> (8, 31) construction
  line L4 (10, 37.5) -> (10, 33) construction
  arc A1 (12, 39.5) -> (10, 37.5) centre (12, 37.5) ccw construction
  line L5 (10.3, 37.5) -> (10.3, 32.9)
  line L6 (-0.3, 32.9) -> (-0.3, 39.1)
  circle A2 centre (5, 36) radius 1.25
  line L7 (-0.3, 32.9) -> (10.3, 32.9)
  line L8 (5, 36) -> (-2.4761, 36) construction
  line L9 (-0.3, 39.1) -> (10.3, 39.1)
  line L10 (10.3, 37.5) -> (10.3, 39.1) construction
  line L11 (-1.8, 39.1) -> (-1.8, 32.9)
  line L12 (-0.3, 39.1) -> (-1.8, 39.1)
  line L13 (-0.3, 32.9) -> (-1.8, 32.9)
  line L14 (10.3, 39.1) -> (10.3, 37.5)
  line L15 (11.8, 39.1) -> (11.8, 32.9)
  line L16 (11.8, 32.9) -> (10.3, 32.9)
  line L17 (11.8, 39.1) -> (10.3, 39.1)
  line L18 (10.3, 37.5) -> (11.8, 37.5)
  line L19 (10, 37.5) -> (12, 37.5) construction
  dimension "d5" = 2.5
  dimension "d7" = 1.5
  dimension "d8" = 1.5
  dimension "d9" = 0.3
  dimension "d10" = 0.3
  dimension "d12" = 6.2
  constraint concentric A0 A2
  constraint parallel L4 L5
  constraint parallel L0 L6
  constraint coincident A0.centre A2.centre
  constraint perpendicular L6 L8
  constraint symmetric L5.end L8 L9.end
  constraint symmetric L6.start L8 L6.end
  constraint parallel L0 L10
  constraint perpendicular L7 L11
  constraint parallel L6 L11
  constraint perpendicular L7 L15
  constraint perpendicular L15 L16
  constraint perpendicular L14 L17
  constraint coincident L15 L18.end
  constraint perpendicular L15 L18
  constraint collinear L9 L12
  constraint collinear L7 L13
  constraint coincident L4.start A1.end
  constraint coincident A1.centre L19.end
  constraint collinear L18 L19
  measures "d5" diameter of A2
  measures "d7" distance of L6 L11
  measures "d8" distance of L5 L15
  measures "d9" distance of L0 L6
  measures "d10" distance of L4 L5
  measures "d12" distance of L7 L9
extrude "Extrude1" add sketch "base" along normal blind 1 contours A2 in component "U64_KeybExt_StandOff"
extrude "Extrude2" add sketch "base" along normal blind 16 contours L5 L6 L7 L9 L14 | L14 L15 L17 L18 in component "U64_KeybExt_StandOff"
extrude "Extrude3" add sketch "base" along normal blind 17.6 contours L5 L15 L16 L18 | L6 L11 L12 L13 in component "U64_KeybExt_StandOff"
fillet "Fillet1" radius 1 4 edges at (11.8, 39.1, 8) (-1.8, 39.1, 8.8) (-1.8, 32.9, 8.8) (11.8, 32.9, 8.8) in component "U64_KeybExt_StandOff"
fillet "Fillet2" radius 0.5 5 edges at (10.3, 37.5, 16.8) (10.3, 32.9, 16.8) (11.8, 37.5, 16.8) (-0.3, 39.1, 16.8) (-0.3, 32.9, 16.8) in component "U64_KeybExt_StandOff"
fillet "Fillet3" radius 0.2 13 edges at (-0.4464, 38.9536, 17.6) (-1.5071, 38.8071, 17.6) (-1.8, 36, 17.6) (-1.5071, 33.1929, 17.6) (-0.4464, 33.0464, 17.6) (-0.3, 36, 17.6) (11.6536, 37.3536, 17.6) (11.05, 37.5, 17.6) (10.4464, 37.3536, 17.6) (10.3, 35.2, 17.6) (10.4464, 33.0464, 17.6) (11.5071, 33.1929, 17.6) (11.8, 35.45, 17.6) in component "U64_KeybExt_StandOff"
fillet "Fillet4" radius 0.2 4 edges at (11.8, 37.55, 16) (11.5071, 38.8071, 16) (5, 39.1, 16) (5, 32.9, 16) in component "U64_KeybExt_StandOff"
component "PCB" placed x (1, 0, 0) y (0, 1, 0) z (0, 0, 1) at (0, 0, 0)
component "U64_KeybExt_StandOff" placed x (1, 0, 0) y (0, 1, 0) z (0, 0, 1) at (0, 0, 0)
equation "d1 = stand_off"
equation "stand_off = 16 mm"
equation "tol = 0.3 mm"
equation "d8 = d7"
equation "d9 = tol"
equation "d10 = tol"
equation "pcb_th = 1.6 mm"
equation "d16 = stand_off"
equation "d18 = stand_off + pcb_th"
equation "filet_out = 1 mm"
equation "d21 = filet_out"
equation "filet_in = 0.5 mm"
equation "d23 = filet_in"
